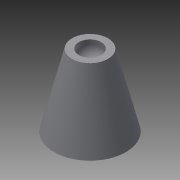
# Autodesk Inventor part: brush fitting
Saved by Autodesk Inventor 2013 SP2 (Build 170200200, 200)
## iProperties
Created: 2017-05-15
Part Number: brush fitting
Material: Generic
Document SubType Name: Modeling
Designer: Herman de Vries
Density: 1 g/cm^3
Author: Herman de Vries
Autodesk Inventor part; units mm, degrees
ref_plane "YZ Plane" through (0, 0, 0) normal (1, 0, 0) x (0, 1, 0)
ref_plane "XZ Plane" through (0, 0, 0) normal (0, 1, 0) x (-1, 0, 0)
ref_plane "XY Plane" through (0, 0, 0) normal (0, 0, 1) x (1, 0, 0)
sketch "Sketch1" plane through (0, 0, 0) normal (1, 0, 0) x (0, 1, 0)
  line L0 (0, 16) -> (4, 16) construction
  arc A0 (7.9892, 0) -> (4, 16) centre (-30.9916, -1.2217) ccw construction
  arc A1 (0, 12.5) -> (2.5, 15) centre (0, 15) ccw
  line L1 (0, 12.5) -> (0, 0) construction
  line L2 (4, 16) -> (2.5, 16)
  line L3 (2.5, 15) -> (2.5, 16)
  line L4 (7.9892, 0) -> (4, 0)
  line L5 (4, 10) -> (0, 10)
  line L6 (4, 10) -> (4, 0)
  line L7 (0, 12.5) -> (0, 10)
  line L8 (7.9892, 0) -> (4, 16)
  dimension "d0" = 4
  dimension "d3" = 5
  dimension "d4" = 1
  dimension "d5" = 4
  dimension "d11" = 10
  dimension "d12" = 16
  dimension "d13" = 104
  constraints: 18 end point, 4 point on circle, 2 centre point, 2 parallel, 2 point on line, 2 vertical, 2 vertical alignment, 1 horizontal, 1 horizontal alignment, 1 perpendicular, 1 tangent
  measures "d0" distance of L0.start L0.end
  measures "d3" diameter of A1
  measures "d4" distance of L0.start A1.centre
  measures "d5" distance of L5.start L5.end
  measures "d11" distance from line of L5 L1.end
  measures "d12" distance from line of L0 L1.end
  measures "d13" angle of L4 L8
revolve "Revolution1" add sketch "Sketch1" angle 360 about axis through (0, 0, 12.5) along (0, 0, -1)
sketch "Sketch2" plane through (0, 0, 0) normal (1, 0, 0) x (0, 1, 0)
  arc A0 (-2.5, 15) -> (2.5, 15) centre (0, 15) ccw projected
  circle A1 centre (0, 15) radius 1.5
  line L0 (0.6744, 16.3398) -> (-0.6744, 13.6602)
  point P0 (0, 0)
  dimension "d8" = 3
  constraints: 2 end point, 2 point on circle, 1 centre point, 1 coincident, 1 midpoint
  measures "d8" diameter of A1
revolve "Revolution2" [suppressed]
body "Solid1"
